tool spacer 20mm (Autodesk Fusion 360 design; units mm, degrees)
Autodesk Fusion 360 part; units mm, degrees
sketch "Sketch1" plane through (0, 0, 0) normal (0, 1, 0) x (1, 0, 0)
  line L0 (0, 0) -> (8, 0)
  line L1 (8, 0) -> (8, -26)
  line L2 (8, -26) -> (0, -26)
  line L3 (0, -26) -> (0, 0)
  dimension "d1" = 8
  dimension "d2" = 26
  constraint horizontal L0
  constraint vertical L1
  constraint horizontal L2
  constraint vertical L3
  constraint coincident L0.start L3.end
  measures "d1" distance of L0.start L0.end
  measures "d2" distance of L0.start L2.end
extrude "Extrude1" add sketch "Sketch1" along normal blind 40 makes body 1
sketch "Sketch2" plane through (8, 0, 0) normal (1, 0, 0) x (0, 0, -1)
  line L0 (-26, 0) -> (0, 0)
  line L1 (0, 0) -> (0, 40)
  line L2 (0, 40) -> (-26, 40)
  line L3 (-26, 40) -> (-26, 0)
  circle A0 centre (-12.7, 20) radius 10
  dimension "d5" = 20
  measures "d5" diameter of A0
extrude "Extrude2" cut sketch "Sketch2" against normal blind 50 contours A0 bodies 1
extrude "Extrude3" cut 1 faces at (2.6667, 40, 8.6667) along direction (0, -1, 0) blind 7 on bodies 1 bodies 1
extrude "Extrude4" cut 1 faces at (2.6667, 0, 8.6667) along direction (0, 1, 0) blind 7 on bodies 1 bodies 1
pattern_linear "R-Pattern1" count 5 spacing 27.5 along (0, 0, 1) count 4 spacing 27 along (0, -1, 0) of bodies 1 makes body 2 at (2.6667, 19.0043, 30.2497) makes body 3 at (2.6667, 19.0043, 57.7497) makes body 4 at (2.6667, 19.0043, 85.2497) makes body 5 at (2.6667, 19.0043, 112.7497) makes body 6 at (2.6667, -7.9957, 2.7497) makes body 7 at (2.6667, -7.9957, 30.2497) makes body 8 at (2.6667, -7.9957, 57.7497) makes body 9 at (2.6667, -7.9957, 85.2497) makes body 10 at (2.6667, -7.9957, 112.7497) makes body 11 at (2.6667, -34.9957, 2.7497) makes body 12 at (2.6667, -34.9957, 30.2497) makes body 13 at (2.6667, -34.9957, 57.7497) makes body 14 at (2.6667, -34.9957, 85.2497) makes body 15 at (2.6667, -34.9957, 112.7497) makes body 16 at (2.6667, -61.9957, 2.7497) makes body 17 at (2.6667, -61.9957, 30.2497) makes body 18 at (2.6667, -61.9957, 57.7497) makes body 19 at (2.6667, -61.9957, 85.2497) makes body 20 at (2.6667, -61.9957, 112.7497)
